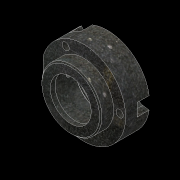
# Autodesk Inventor part: KON_Nietmaschine_Deckel
Saved by Autodesk Inventor 2019 (Build 230136000, 136)
## iProperties
Created: 2022-01-03
Part Number: KON_Nietmaschine_Deckel
Material: Stahl
Document SubType Name: Modeling
Designer: Jonas Nebl
Density: 7.85 g/cm^3
Appearance: Platte
Mass: 420.867 g
Surface Area: 173.325 cm^2
Volume: 53.6137 cm^3
Author: Jonas Nebl
Autodesk Inventor part; units mm, degrees
ref_plane "XZ Plane" through (0, 0, 0) normal (0, 1, 0) x (-1, 0, 0)
ref_plane "XY Plane" through (0, 0, 0) normal (0, 0, 1) x (1, 0, 0)
sketch "Skizze1" plane through (0, 0, 0) normal (0, 1, 0) x (-1, 0, 0)
  line L0 (17, 30.75) -> (17, 26.75)
  line L1 (17, 26.75) -> (20, 26.75)
  line L2 (20, 26.75) -> (20, 6.75)
  line L3 (23, 0) -> (35, 0)
  line L4 (35, 0) -> (35, 20)
  line L5 (35, 20) -> (25, 20)
  line L6 (25, 20) -> (25, 30.75)
  line L7 (17, 30.75) -> (25, 30.75)
  line L8 (0, 0) -> (0, 48.4152)
  line L9 (20, 6.75) -> (23, 6.75)
  line L10 (23, 6.75) -> (23, 4.75)
  line L11 (23, 4.75) -> (25, 4.75)
  line L12 (25, 4.75) -> (25, 3)
  line L13 (25, 3) -> (23, 3)
  line L14 (23, 3) -> (23, 0)
  point P0 (17, 4)
  dimension "d1" = 40
  dimension "d3" = 20
  dimension "d4" = 70
  dimension "d5" = 50
  dimension "d7" = 4
  dimension "d10" = 2
  dimension "d11" = 1.75
  dimension "d12" = 3
  dimension "d13" = 3
  dimension "d14" = 2
  dimension "d15" = 34
  dimension "d16" = 20
  constraints: 31 end point, 8 vertical, 7 horizontal, 3 point on line
  measures "d1" diameter of L2 L8
  measures "d3" distance of L3.end L4.end
  measures "d4" diameter of L4 L8
  measures "d5" diameter of L6 L8
  measures "d7" distance between parallel lines of L1 L7
  measures "d10" distance of L9.end L10.end
  measures "d11" distance of L11.end L12.end
  measures "d12" distance of L13.end L3.start
  measures "d13" distance of L2.end L9.end
  measures "d14" distance of L12.end L13.end
  measures "d15" diameter of L0 L8
  measures "d16" distance of L1.end L2.end
revolve "Umdrehung1" add sketch "Skizze1" angle 360 about axis through (0, 0, 0) along (0, 0, 1)
sketch "Skizze2" plane through (0, 0, 0) normal (0, 0, -1) x (-1, 0, 0)
  circle A0 centre (0, 0) radius 23 projected
  circle A1 centre (0, 0) radius 35 projected
  arc A2 (-29.325, -4.4491) -> (-29.325, 4.4491) centre (-30, 0) ccw
  line L0 (-29.325, 4.4491) -> (-34.604, 5.25)
  line L1 (-29.325, -4.4491) -> (-34.604, -5.25)
  line L2 (49, 0) -> (-49, 0) projected
  line L3 (10.8095, -27.6207) -> (12.7554, -32.593)
  arc A3 (18.5155, -23.1717) -> (10.8095, -27.6207) centre (15, -25.9808) ccw
  line L4 (18.5155, -23.1717) -> (21.8486, -27.343)
  line L5 (18.5155, 23.1717) -> (21.8486, 27.343)
  arc A4 (10.8095, 27.6207) -> (18.5155, 23.1717) centre (15, 25.9808) ccw
  line L6 (10.8095, 27.6207) -> (12.7554, 32.593)
  arc A5 (21.8486, 27.343) -> (12.7554, 32.593) centre (0, 0) ccw
  arc A6 (12.7554, -32.593) -> (21.8486, -27.343) centre (0, 0) ccw
  arc A7 (-34.604, 5.25) -> (-34.604, -5.25) centre (0, 0) ccw
  dimension "d17" = 30
  dimension "d18" = 4.5
  dimension "d21" = 360
  constraints: 14 point on circle, 12 end point, 6 centre point, 4 coincident, 2 line through centre, 2 tangent, 1 point on line, 29 other
  measures "d17" distance of A2.centre A1.centre
  measures "d18" radius of A2
extrude "Extrusion1" cut sketch "Skizze2" against normal blind 10 contours L2 A1 L0 A2 | A2 L1 A1 L2 | L5 A4 L6 A1 | A1 L3 A3 L4
sketch "Skizze3" plane through (0, 0, 0) normal (0, 0, -1) x (-1, 0, 0)
  arc A0 (10.8095, 27.6207) -> (18.5155, 23.1717) centre (15, 25.9808) ccw projected
  arc A1 (-29.325, -4.4491) -> (-29.325, 4.4491) centre (-30, 0) ccw projected
  arc A2 (18.5155, -23.1717) -> (10.8095, -27.6207) centre (15, -25.9808) ccw projected
  point P0 (-30, 0)
  point P1 (15, 25.9808)
  point P2 (15, -25.9808)
  constraints: 3 coincident
hole "Bohrung1" at (30, 0, 0) at (-15, 25.9808, 0) at (-15, -25.9808, 0) direction (0, 0, 1) diameter 6 end through all
ref_plane "Arbeitsebene1" through (-40, 0, 0) normal (1, 0, 0) x (0, 1, 0)
sketch "Skizze4" plane through (-40, 0, 0) normal (1, 0, 0) x (0, 1, 0)
  line L0 (-25, 20) -> (25, 20) projected
  line L1 (10, 20) -> (-10, 20)
  line L2 (-10, 20) -> (-10, 0)
  line L3 (-10, 0) -> (10, 0)
  line L4 (10, 0) -> (10, 20)
  line L5 (-27.343, 0) -> (27.343, 0) projected
  line L6 (0, -4) -> (0, 24) projected
  point P0 (0, 0)
  constraints: 8 end point, 2 parallel, 2 perpendicular, 2 point on line, 1 horizontal, 1 other
extrude "Extrusion2" cut sketch "Skizze4" along normal blind 6.4
sketch "Skizze5" plane through (-33.6, 0, 0) normal (-1, 0, 0) x (0, 0, 1)
  line L0 (-6.15, 0) -> (36.9, 0) projected
  line L1 (0, -9.8) -> (0, 9.8) projected
  point P0 (0, 0)
  point P1 (12, 0)
  dimension "d47" = 12
  constraints: 1 point on line
  measures "d47" distance from line of point (12, 0) L1
hole "Bohrung2" at (-33.6, 0, 12) direction (1, 0, 0) diameter 5 depth 20 tip angle 118
thread "Gewinde1" size "M6x1" class "6H" standard "ISO Metric profile" full length
chamfer "Fase1" distance 1 angle 45 1 edges at (25, 0, 30.75)
